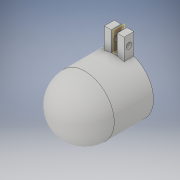
# Autodesk Inventor part: beta_dummy _thumb
Saved by Autodesk Inventor 2018 (Build 220112000, 112)
## iProperties
Created: 2017-10-07
Part Number: beta_dummy _thumb
Material: Generic
Document SubType Name: Modeling
Designer: rheal
Density: 1 g/cm^3
Appearance: Default
Author: rheal
Autodesk Inventor part; units mm, degrees
ref_plane "YZ Plane" through (0, 0, 0) normal (1, 0, 0) x (0, 1, 0)
ref_plane "XZ Plane" through (0, 0, 0) normal (0, 1, 0) x (-1, 0, 0)
ref_plane "XY Plane" through (0, 0, 0) normal (0, 0, 1) x (1, 0, 0)
sketch "Sketch1" plane through (0, 0, 0) normal (0, 0, 1) x (1, 0, 0)
  line L0 (-5, 20) -> (-5, 9.1421)
  line L1 (0, 10) -> (0, 17.0552) construction
  line L2 (5, 20) -> (5, 9.1421)
  line L3 (5, 10) -> (-5, 10) construction
  line L4 (0, 10) -> (0, 20) construction
  line L5 (-1.5, 20) -> (-1.5, 10)
  line L6 (1.5, 20) -> (1.5, 10)
  line L7 (5, 20) -> (1.5, 20)
  line L8 (-1.5, 20) -> (-5, 20)
  line L9 (-1.5, 10) -> (1.5, 10)
  arc A0 (-5, 9.1421) -> (5, 9.1421) centre (0, -5) ccw
  circle A1 centre (0, -5) radius 12.5
  dimension "d46" = 1.5
  dimension "d61" = 25
  constraints: 20 end point, 3 perpendicular, 3 point on line, 3 vertical, 2 centre point, 2 point on circle, 2 symmetric about line, 1 coincident, 1 collinear, 1 horizontal, 1 tangent
  measures "d46" distance of L4.end L5.start
  measures "d61" diameter of A1
extrude "Extrusion1" add sketch "Sketch1" along normal blind 5
sketch "Sketch4" plane through (5, 5.9087, 0) normal (1, 0, 0) x (0, 0, -1)
  line L0 (0, 14.0913) -> (-5, 14.0913) construction
  line L1 (-2.5, 14.0913) -> (-2.5, 9.0913) construction
  circle A0 centre (-2.5, 9.0913) radius 1.5
  point P0 (0, -5.9087)
  dimension "d30" = 5
  dimension "d31" = 3
  constraints: 2 end point, 1 centre point, 1 coincident, 1 midpoint, 1 vertical
  measures "d30" distance of L1.start L1.end
  measures "d31" diameter of A0
extrude "Extrusion4" cut sketch "Sketch4" against normal blind 10
ref_plane "Work Plane1" through (0, 5.9087, 0) normal (1, 0, 0) x (0, 0, -1)
ref_plane "Work Plane2" through (0, 5.9087, 0) normal (1, 0, 0) x (0, 0, -1)
sketch "Sketch14" plane through (0, 5.9087, 0) normal (1, 0, 0) x (0, 0, -1)
  line L0 (-5, 1.5913) -> (-20, 1.5913)
  line L1 (-20, 1.5913) -> (-20, 4.0913)
  line L2 (-20, 4.0913) -> (-5, 4.0913)
  line L3 (-5, 1.5913) -> (-5, -23.4087) construction
  line L4 (-5, -10.9087) -> (-20, -10.9087) construction
  line L5 (-5, -23.4087) -> (-5, 1.5913) projected
  line L6 (-5, 4.0913) -> (-5, 1.5913)
  point P0 (0, -5.9087)
  dimension "d62" = 15
  dimension "d63" = 2.5
  dimension "d64" = 15
  constraints: 12 end point, 3 perpendicular, 2 horizontal, 1 midpoint, 1 vertical
  measures "d62" distance of L0.start L0.end
  measures "d63" distance of L0.end L1.end
  measures "d64" distance of L4.start L4.end
revolve "Revolution3" add sketch "Sketch14" angle 360 about axis through (0, -5, 5) along (0, 0, 1)
sketch "Sketch15" plane through (0, 5.9087, 0) normal (1, 0, 0) x (0, 0, -1)
  line L0 (-20, -23.4087) -> (-20, 1.5913) projected
  arc A0 (-20, 1.5913) -> (-32.5, -10.9087) centre (-20, -10.9087) ccw
  arc A1 (-20, 4.0913) -> (-35, -10.9087) centre (-20, -10.9087) ccw
  line L1 (-32.5, -10.9087) -> (-35, -10.9087) construction
  line L2 (-20, 1.5913) -> (-20, -23.4087) construction
  line L3 (-20, -25.9087) -> (-20, 4.0913) projected
  line L4 (-20, 1.5913) -> (-20, 4.0913)
  line L5 (-32.5, -10.9087) -> (-35, -10.9087)
  point P0 (0, -5.9087)
  dimension "d67" = 30
  constraints: 9 end point, 4 point on circle, 2 centre point, 2 horizontal, 1 coincident, 1 perpendicular, 1 point on line, 1 vertical
  measures "d67" diameter of A1
revolve "Revolution4" add sketch "Sketch15" angle 360 about axis through (0, -5, 32.5) along (0, 0, 1)
body "Solid1"
